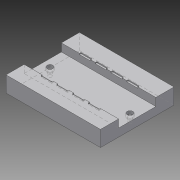
# Autodesk Inventor part: UNLHEP-14-01-P-016_StampStoragePlate
Saved by Autodesk Inventor 2013 (Build 170138000, 138)
## iProperties
Created: 2014-01-23
Part Number: UNLHEP-14-01-P-016_StampStoragePlate
Material: Allgemein
Document SubType Name: Modeling
Designer: Frank Meier
Density: 1 g/cm^3
Author: Frank Meier
Autodesk Inventor part; units mm, degrees
ref_plane "YZ Plane" through (0, 0, 0) normal (1, 0, 0) x (0, 1, 0)
ref_plane "XZ Plane" through (0, 0, 0) normal (0, 1, 0) x (-1, 0, 0)
ref_plane "XY Plane" through (0, 0, 0) normal (0, 0, 1) x (1, 0, 0)
sketch "Skizze1" plane through (0, 0, 0) normal (0, 0, 1) x (1, 0, 0)
  line L0 (-90, -70) -> (90, -70)
  line L1 (90, -70) -> (90, 70)
  line L2 (90, 70) -> (-90, 70)
  line L3 (-90, 70) -> (-90, -70)
  line L4 (-90, -70) -> (90, 70) construction
  line L5 (90, -70) -> (-90, 70) construction
  point P0 (0, 0)
  dimension "d0" = 180
  dimension "d1" = 140
  constraints: 12 end point, 2 midpoint, 2 parallel, 1 horizontal, 1 perpendicular
  measures "d0" distance of L1.end L2.end
  measures "d1" distance of L0.end L1.end
extrude "Extrusion1" add sketch "Skizze1" along normal blind 30
sketch "Skizze3" plane through (90, -70, 0) normal (1, 0, 0) x (0, 0, -1)
  line L0 (-30, 0) -> (-30, 140) projected
  line L1 (0, 0) -> (-30, 0) projected
  line L2 (-30, 34.5) -> (-15, 34.5)
  line L3 (-15, 34.5) -> (-15, 105.5)
  line L4 (-15, 105.5) -> (-30, 105.5)
  line L5 (-30, 105.5) -> (-30, 34.5)
  point P0 (0, 70)
  dimension "d6" = 71
  dimension "d7" = 15
  dimension "d8" = 34.5
  constraints: 8 end point, 2 parallel, 1 horizontal, 1 perpendicular, 1 point on line
  measures "d6" distance of L4.end L2.start
  measures "d7" distance of L3.end L4.end
  measures "d8" distance between parallel lines of L1 L2
extrude "Extrusion2" cut sketch "Skizze3" against normal blind 180
sketch "Skizze4" plane through (0, 0, 30) normal (0, 0, 1) x (1, 0, 0)
  line L0 (90, -35.5) -> (-90, -35.5) projected
  line L1 (-90, -70) -> (90, -70) projected
  line L2 (-90, -70) -> (90, -70) projected
  line L3 (-90, 70) -> (-90, -70) projected
  line L4 (90, 70) -> (-90, 70) projected
  line L5 (90, -70) -> (90, 70) projected
  line L6 (-55.5, -38.5) -> (-34.5, -38.5)
  line L7 (-34.5, -38.5) -> (-34.5, 38.5)
  line L8 (-34.5, 38.5) -> (-55.5, 38.5)
  line L9 (-55.5, 38.5) -> (-55.5, -38.5)
  line L10 (-55.5, -38.5) -> (-34.5, 38.5) construction
  line L11 (-34.5, -38.5) -> (-55.5, 38.5) construction
  line L12 (-25.5, -38.5) -> (-4.5, -38.5)
  line L13 (-4.5, -38.5) -> (-4.5, 38.5)
  line L14 (-4.5, 38.5) -> (-25.5, 38.5)
  line L15 (-25.5, 38.5) -> (-25.5, -38.5)
  line L16 (-25.5, -38.5) -> (-4.5, 38.5) construction
  line L17 (-4.5, -38.5) -> (-25.5, 38.5) construction
  line L18 (4.5, -38.5) -> (25.5, -38.5)
  line L19 (25.5, -38.5) -> (25.5, 38.5)
  line L20 (25.5, 38.5) -> (4.5, 38.5)
  line L21 (4.5, 38.5) -> (4.5, -38.5)
  line L22 (4.5, -38.5) -> (25.5, 38.5) construction
  line L23 (25.5, -38.5) -> (4.5, 38.5) construction
  line L24 (34.5, -38.5) -> (55.5, -38.5)
  line L25 (55.5, -38.5) -> (55.5, 38.5)
  line L26 (55.5, 38.5) -> (34.5, 38.5)
  line L27 (34.5, 38.5) -> (34.5, -38.5)
  line L28 (34.5, -38.5) -> (55.5, 38.5) construction
  line L29 (55.5, -38.5) -> (34.5, 38.5) construction
  point P0 (0, 0)
  point P1 (-45, 0)
  point P2 (-15, 0)
  point P3 (15, 0)
  point P4 (45, 0)
  point P5 (-50, -35.5)
  dimension "d11" = 21
  dimension "d12" = 77
  dimension "d13" = 3
  dimension "d14" = 34.5
  dimension "d17" = 30
  constraints: 48 end point, 8 midpoint, 2 horizontal, 2 parallel, 1 perpendicular, 33 other
  measures "d11" distance of L7.end L8.end
  measures "d12" distance of L6.end L7.end
  measures "d13" distance between parallel lines of L0 L6
  measures "d14" distance between parallel lines of L3 L9
  measures "d17" distance of L6.start L12.start
extrude "Extrusion3" cut sketch "Skizze4" against normal blind 2 contours L25 L24 L27 L0 | L0 L27 L26 L25 | L19 L18 L21 L0 | L0 L21 L20 L19 | L9 L8 L7 L0 | L0 L7 L6 L9 | L13 L12 L15 L0 | L0 L15 L14 L13
fillet "Rundung1" radius 1 1 edges at (-55.5, 38.5, 29)
fillet "Rundung2" radius 1 15 edges at (-25.5, 38.5, 29) (4.5, 38.5, 29) (-4.5, 38.5, 29) (25.5, 38.5, 29) (34.5, 38.5, 29) (55.5, 38.5, 29) (-34.5, 38.5, 29) (-55.5, -38.5, 29) (-34.5, -38.5, 29) (-25.5, -38.5, 29) (-4.5, -38.5, 29) (4.5, -38.5, 29) (25.5, -38.5, 29) (34.5, -38.5, 29) (55.5, -38.5, 29)
sketch "Skizze5" plane through (90, -35.5, 15) normal (0, 0, 1) x (1, 0, 0)
  line L0 (0, 71) -> (0, 0) projected
  point P0 (-90, 35.5)
  point P1 (-166.2, 35.5)
  point P2 (-13.8, 35.5)
  dimension "d26" = 152.4
  dimension "d28" = 13.8
  measures "d26" distance of point (-13.8, 35.5) point (-166.2, 35.5)
  measures "d28" distance from line of L0 point (-13.8, 35.5)
hole "Bohrung1" at (-76.2, 0, 15) at (76.2, 0, 15) direction (0, 0, -1) diameter 6.756 depth 20 tip angle 118 counterbore diameter 11.113 counterbore depth 6.35 clearance for "Innensechskantkopfschraube" size "1/4" standard "ANSI UST"
